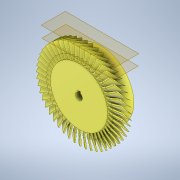
# Autodesk Inventor part: Rotor.48.2.6
Saved by Autodesk Inventor 2021.2 (Build 252289000, 289)
## iProperties
Created: 2021-05-16
Part Number: Rotor.48.2.6
Material: Generic
Document SubType Name: Modeling
Designer: Ryan
Density: 1 g/cm^3
Appearance: Smooth - Yellow
Author: Ryan
## iProperties of the stored document _3DPrint.ipt
Created: 2021-05-17
Part Number: _3DPrint
Material: Generic
Document SubType Name: Modeling
Designer: Ryan
Density: 1 g/cm^3
Appearance: Default
Author: Ryan
Autodesk Inventor part; units mm, degrees
ref_plane "YZ Plane" through (0, 0, 0) normal (1, 0, 0) x (0, 1, 0)
ref_plane "XY Plane" through (0, 0, 0) normal (0, 0, 1) x (1, 0, 0)
sketch "Sketch1" plane through (0, 0, 0) normal (0, 0, 1) x (1, 0, 0)
  circle A0 centre (0, 0) radius 33.02
  dimension "d0" = 66.04
  constraints: 1 centre point, 1 coincident
  measures "d0" diameter of A0
extrude "Extrusion1" add sketch "Sketch1" against normal blind 25.4 draft 11.31
ref_plane "Work Plane1" through (0, 38.1, 0) normal (0, 1, 0) x (-1, 0, 0)
sketch "Sketch2" plane through (0, 38.1, 0) normal (0, 1, 0) x (-1, 0, 0)
  arc A0 (5.6212, -1.563) -> (4.774, -0.1017) centre (5.1759, -0.8449) ccw
  line L0 (33.02, 0) -> (38.1, -25.4) projected
  line L1 (35.56, -12.7) -> (18.0568, -12.7)
  line L2 (33.02, 0) -> (-33.02, 0) projected
  arc A1 (4.774, -0.1017) -> (-3.0859, -11.9063) centre (12.9535, -14.0669) ccw
  arc A2 (5.6212, -1.563) -> (-3.0859, -11.9063) centre (15.1085, -18.3861) ccw
  point P0 (0, 0)
  dimension "d4" = 0.7937
  constraints: 6 point on circle, 3 centre point, 2 end point, 1 horizontal, 1 midpoint, 1 tangent
  measures "d4" distance from line of A1.end L1
extrude "Extrusion2" add sketch "Sketch2" against normal blind 12.7
ref_plane "Work Plane2" through (0, 50.8, 0) normal (0, 1, 0) x (-1, 0, 0)
sketch "Sketch4" plane through (0, 50.8, 0) normal (0, 1, 0) x (-1, 0, 0)
  arc A0 (7.5472, -1.6631) -> (6.8775, -0.6716) centre (7.1887, -1.1833) ccw
  arc A1 (6.8775, -0.6716) -> (-5.2339, -11.3184) centre (30.9975, -40.3215) ccw
  arc A2 (7.5472, -1.6631) -> (-5.2339, -11.3184) centre (30.972, -45.9588) ccw
  point P0 (0, 0)
  constraints: 6 point on circle, 3 centre point
loft "Loft3" add profiles "Sketch4" section 2 edges at (0.5178, 38.1, -5.0972) (-0.333, 38.1, -5.9478) (-5.9068, 38.1, -0.4211)
pattern_circular "Circular Pattern6" count 48 over 360 about axis through (0, 0, 0) along (0, 0, -1) of "Loft3", "Extrusion2"
sketch "Sketch5" plane through (0, 0, 0) normal (0, 0, 1) x (1, 0, 0)
  circle A0 centre (0, 0) radius 4
  line L0 (-1.5875, 5.5875) -> (1.5875, 5.5875)
  line L1 (1.5875, 5.5875) -> (1.5875, 2.4125)
  line L2 (1.5875, 2.4125) -> (-1.5875, 2.4125)
  line L3 (-1.5875, 2.4125) -> (-1.5875, 5.5875)
  line L4 (-1.5875, 5.5875) -> (1.5875, 2.4125) construction
  line L5 (1.5875, 5.5875) -> (-1.5875, 2.4125) construction
  point P0 (0, 4)
  point P1 (-1.5875, 3.6715)
  point P2 (1.5875, 3.6715)
  dimension "d38" = 8
  dimension "d39" = 3.175
  dimension "d40" = 3.175
  constraints: 12 end point, 2 midpoint, 2 parallel, 1 coincident, 1 horizontal, 1 perpendicular, 3 other
  measures "d39" distance of L1.end L2.end
  measures "d40" distance of L0.end L1.end
extrude "Extrusion3" cut sketch "Sketch5" against normal through all
sketch "Sketch6" plane through (0, 0, 0) normal (0, 0, 1) x (1, 0, 0)
  circle A0 centre (0, 0) radius 50.0063
  circle A1 centre (0, 0) radius 81.7071
  dimension "d43" = 100.0125
  constraints: 2 centre point, 2 coincident
  measures "d43" diameter of A0
extrude "Extrusion4" cut sketch "Sketch6" against normal through all
body "Solid1"
